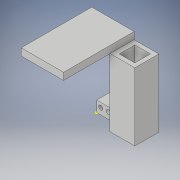
# Autodesk Inventor part: servo_rack
Saved by Autodesk Inventor 2018.1 (Build 221171000, 171)
## iProperties
Created: 2017-11-15
Part Number: servo_rack
Material: Generic
Document SubType Name: Modeling
Designer: bramd
Density: 1 g/cm^3
Appearance: Default
Author: bramd
Autodesk Inventor part; units mm, degrees
ref_plane "YZ Plane" through (0, 0, 0) normal (1, 0, 0) x (0, 1, 0)
ref_plane "XZ Plane" through (0, 0, 0) normal (0, 1, 0) x (-1, 0, 0)
ref_plane "XY Plane" through (0, 0, 0) normal (0, 0, 1) x (1, 0, 0)
sketch "Sketch1" plane through (0, 0, 0) normal (0, 0, 1) x (1, 0, 0)
  line L0 (0, 0) -> (70.612, 0)
  line L1 (70.612, 0) -> (70.612, 60.96)
  line L2 (70.612, 60.96) -> (0, 60.96)
  line L3 (0, 60.96) -> (0, 0)
  dimension "d0" = 70.612
  dimension "d1" = 60.96
  constraints: 8 end point, 2 parallel, 1 horizontal, 1 perpendicular
  measures "d0" distance of L1.end L2.end
  measures "d1" distance of L2.end L0.start
sketch "Sketch2" plane through (0, 0, 0) normal (0, 0, 1) x (1, 0, 0)
  point P0 (0, 0)
extrude "Extrusion1" add sketch "Sketch1" along normal blind 12.7
sketch "Sketch3" plane through (0, 0, 12.7) normal (0, 0, 1) x (1, 0, 0)
  circle A0 centre (3.683, 54.61) radius 1.905
  circle A1 centre (10.541, 54.61) radius 1.905
  circle A2 centre (3.683, 5.715) radius 1.905
  circle A3 centre (10.541, 5.715) radius 1.905
  point P0 (0, 0)
  dimension "d4" = 3.81
  dimension "d5" = 3.81
  dimension "d6" = 3.81
  dimension "d7" = 3.81
  constraints: 4 centre point
  measures "d4" diameter of A1
  measures "d5" diameter of A0
  measures "d6" diameter of A3
  measures "d7" diameter of A2
extrude "Extrusion2" cut sketch "Sketch3" against normal blind 12.7
sketch "Sketch4" plane through (0, 0, 12.7) normal (0, 0, 1) x (1, 0, 0)
  line L0 (70.612, 60.96) -> (0, 60.96) projected
  line L1 (70.612, 0) -> (70.612, 60.96) projected
  line L2 (38.1, 60.96) -> (70.612, 60.96)
  line L3 (70.612, 60.96) -> (70.612, 0)
  line L4 (70.612, 0) -> (38.1, 0)
  line L5 (38.1, 0) -> (38.1, 60.96)
  line L6 (0, 60.96) -> (0, 0) projected
  dimension "d10" = 38.1
  constraints: 8 end point, 2 parallel, 1 horizontal, 1 perpendicular, 1 point on line
  measures "d10" distance between parallel lines of L5 L6
extrude "Extrusion3" add sketch "Sketch4" along normal blind 20.32
sketch "Sketch5" plane through (0, 0, 12.7) normal (0, 0, 1) x (1, 0, 0)
  line L0 (0, 60.96) -> (0, 0) projected
  line L1 (0, 9.8425) -> (20.955, 9.8425)
  line L2 (20.955, 9.8425) -> (20.955, 50.4825)
  line L3 (20.955, 50.4825) -> (0, 50.4825)
  line L4 (0, 50.4825) -> (0, 9.8425)
  dimension "d13" = 20.955
  dimension "d14" = 40.64
  constraints: 8 end point, 2 parallel, 1 horizontal, 1 perpendicular, 1 point on line
  measures "d13" distance of L3.end L2.end
  measures "d14" distance of L2.end L1.end
extrude "Extrusion4" cut sketch "Sketch5" against normal blind 12.7
sketch "Sketch6" plane through (0, 60.96, 0) normal (0, 1, 0) x (1, 0, 0)
  line L0 (12.446, -12.7) -> (12.446, 0) projected
  line L1 (12.446, 0) -> (53.086, 0)
  line L2 (53.086, 0) -> (53.086, -12.7)
  line L3 (53.086, -12.7) -> (12.446, -12.7)
  line L4 (12.446, -12.7) -> (12.446, 0)
  point P0 (0, 0)
  dimension "d17" = 40.64
  constraints: 8 end point, 2 parallel, 1 horizontal, 1 perpendicular, 1 point on line
  measures "d17" distance of L2.end L3.end
extrude "Extrusion5" add sketch "Sketch6" along normal blind 20.32
sketch "Sketch7" plane through (0, 0, 12.7) normal (0, 0, 1) x (1, 0, 0)
  circle A0 centre (20.955, 76.2) radius 1.905
  circle A1 centre (20.955, 67.31) radius 1.905
  circle A2 centre (40.64, 67.31) radius 1.905
  circle A3 centre (40.64, 76.2) radius 1.905
  point P0 (0, 0)
  dimension "d20" = 3.81
  dimension "d21" = 3.81
  dimension "d22" = 3.81
  dimension "d23" = 3.81
  constraints: 4 centre point
  measures "d20" diameter of A0
  measures "d21" diameter of A1
  measures "d22" diameter of A2
  measures "d23" diameter of A3
extrude "Extrusion6" cut sketch "Sketch7" against normal blind 12.7
sketch "Sketch8" plane through (0, 0, 12.7) normal (0, 0, 1) x (1, 0, 0)
  line L0 (12.446, 60.96) -> (12.446, 81.28) projected
  line L1 (70.612, 60.96) -> (53.086, 60.96) projected
  line L2 (12.446, 81.28) -> (53.086, 81.28)
  line L3 (53.086, 81.28) -> (53.086, 60.96)
  line L4 (53.086, 60.96) -> (12.446, 60.96)
  line L5 (12.446, 60.96) -> (12.446, 81.28)
  point P0 (0, 0)
  constraints: 8 end point, 2 parallel, 1 horizontal, 1 perpendicular
extrude "Extrusion7" cut sketch "Sketch8" against normal blind 25.4
sketch "Sketch9" plane through (0, 0, 12.7) normal (0, 0, 1) x (1, 0, 0)
  point P0 (0, 0)
sketch "Sketch10" plane through (0, 0, 33.02) normal (0, 0, 1) x (1, 0, 0)
  line L0 (38.1, 60.96) -> (0, 60.96) projected
  line L1 (38.1, 0) -> (20.7539, 0)
  line L2 (20.7539, 0) -> (20.7539, 60.96)
  line L3 (20.7539, 60.96) -> (38.1, 60.96)
  line L4 (38.1, 60.96) -> (38.1, 0)
  point P0 (0, 0)
  constraints: 8 end point, 2 parallel, 1 horizontal, 1 perpendicular, 1 point on line
extrude "Extrusion8" add sketch "Sketch10" against normal blind 20.32
sketch "Sketch11" plane through (0, 0, 0) normal (0, -1, 0) x (1, 0, 0)
  line L0 (70.612, 33.02) -> (20.7539, 33.02) projected
  line L1 (0, 0) -> (70.612, 0) projected
  line L2 (70.612, 33.02) -> (45.212, 33.02)
  line L3 (45.212, 33.02) -> (45.212, 0)
  line L4 (45.212, 0) -> (70.612, 0)
  line L5 (70.612, 0) -> (70.612, 33.02)
  dimension "d30" = 25.4
  constraints: 8 end point, 2 parallel, 1 horizontal, 1 perpendicular, 1 point on line
  measures "d30" distance of L4.end L3.end
extrude "Extrusion9" cut sketch "Sketch11" against normal blind 76.2
sketch "Sketch12" plane through (0, 0, 0) normal (0, -1, 0) x (1, 0, 0)
  line L0 (25.4, 3.81) -> (39.37, 3.81)
  line L1 (39.37, 3.81) -> (39.37, 17.78)
  line L2 (39.37, 17.78) -> (25.4, 17.78)
  line L3 (25.4, 17.78) -> (25.4, 3.81)
  point P0 (0, 0)
  dimension "d33" = 13.97
  dimension "d34" = 13.97
  constraints: 8 end point, 2 parallel, 1 horizontal, 1 perpendicular
  measures "d33" distance of L2.end L1.end
  measures "d34" distance of L1.end L0.end
extrude "Extrusion10" cut sketch "Sketch12" against normal blind 76.2
sketch "Sketch13" plane through (0, 0, 0) normal (0, -1, 0) x (1, 0, 0)
  line L0 (20.7539, 33.02) -> (20.7539, 12.7) projected
  line L1 (45.212, 33.02) -> (20.7539, 33.02) projected
  line L2 (20.7539, 21.59) -> (45.212, 21.59)
  line L3 (45.212, 21.59) -> (45.212, 33.02)
  line L4 (45.212, 33.02) -> (20.7539, 33.02)
  line L5 (20.7539, 33.02) -> (20.7539, 21.59)
  point P0 (0, 0)
  constraints: 8 end point, 2 parallel, 1 horizontal, 1 perpendicular, 1 point on line
extrude "Extrusion11" cut sketch "Sketch13" against normal blind 76.2
sketch "Sketch14" plane through (0, 60.96, 12.7) normal (0, 1, 0) x (1, 0, 0)
  line L0 (45.212, -8.89) -> (20.7539, -8.89) projected
  line L1 (45.212, -8.89) -> (43.18, -8.89)
  line L2 (43.18, -8.89) -> (43.18, 12.7)
  line L3 (43.18, 12.7) -> (45.212, 12.7)
  line L4 (45.212, 12.7) -> (45.212, -8.89)
  point P0 (0, 12.7)
  dimension "d39" = 2.032
  constraints: 8 end point, 2 parallel, 1 horizontal, 1 perpendicular
  measures "d39" distance of L2.end L3.end
extrude "Extrusion12" cut sketch "Sketch14" against normal blind 76.2
sketch "Sketch15" plane through (0, 60.96, 12.7) normal (0, 1, 0) x (1, 0, 0)
  line L0 (20.955, 0) -> (20.955, 12.7) projected
  line L1 (20.955, 12.7) -> (-17.145, 12.7)
  line L2 (-17.145, 12.7) -> (-17.145, -50.8)
  line L3 (-17.145, -50.8) -> (20.955, -50.8)
  line L4 (20.955, -50.8) -> (20.955, 12.7)
  point P0 (0, 12.7)
  dimension "d42" = 38.1
  dimension "d43" = 63.5
  constraints: 8 end point, 2 parallel, 1 horizontal, 1 perpendicular
  measures "d42" distance of L3.end L2.end
  measures "d43" distance of L2.end L1.end
extrude "Extrusion13" add sketch "Sketch15" along normal blind 6.35
body "Solid1"
